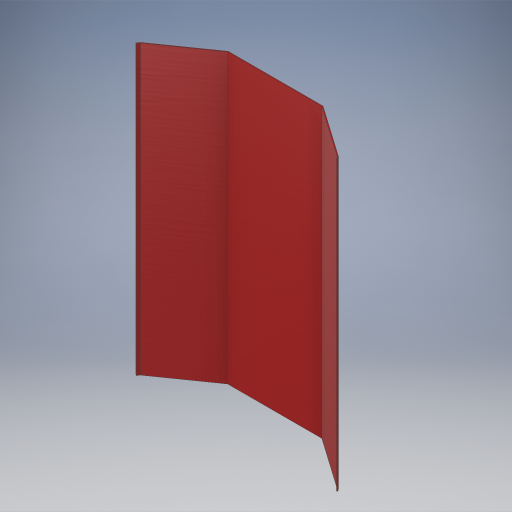
# Autodesk Inventor part: Gummi Matte
Saved by Autodesk Inventor 2023.2 (Build 272271000, 271)
## iProperties
Created: 2023-02-05
Part Number: Gummi Matte
Material: Gummi
Document SubType Name: Modeling
Designer: Raoul Messerli
Density: 0.93 g/cm^3
Appearance: Gummi - Schwarz
Author: Raoul Messerli
Autodesk Inventor part; units mm, degrees
ref_plane "YZ Plane" through (0, 0, 0) normal (1, 0, 0) x (0, 1, 0)
ref_plane "XZ Plane" through (0, 0, 0) normal (0, 1, 0) x (-1, 0, 0)
ref_plane "XY Plane" through (0, 0, 0) normal (0, 0, 1) x (1, 0, 0)
sketch "Skizze1" plane through (0, 0, 0) normal (0, 0, 1) x (1, 0, 0)
  line L0 (0, 0) -> (148.3505, 0)
  line L1 (0, 0) -> (-148.3505, 0)
  line L2 (-148.3505, 0) -> (-310.097, -113.2561)
  line L3 (148.3505, 0) -> (310.097, -113.2561)
  line L4 (310.097, -113.2561) -> (315.8328, -121.4476)
  line L5 (-310.097, -113.2561) -> (-315.8328, -121.4476)
  line L6 (-313.3753, -123.1684) -> (-307.9429, -115.4102)
  line L7 (-307.9429, -115.4102) -> (-147.4046, -3)
  line L8 (-147.4046, -3) -> (0, -3)
  line L9 (0, -3) -> (147.4046, -3)
  line L10 (147.4046, -3) -> (307.9429, -115.4102)
  line L11 (307.9429, -115.4102) -> (313.3753, -123.1684)
  line L12 (-315.8328, -121.4476) -> (-313.3753, -123.1684)
  line L13 (315.8328, -121.4476) -> (313.3753, -123.1684)
  dimension "d0" = 145
  dimension "d1" = 160
  dimension "d2" = 145
  dimension "d3" = 160
  dimension "d4" = 197.456
  dimension "d5" = 296.701
  dimension "d6" = 10
  dimension "d7" = 3
  constraints: 28 end point, 3 equal length, 2 horizontal, 5 other
  measures "d0" angle of L1 L2
  measures "d1" angle of L2 L5
  measures "d2" angle of L3 L0
  measures "d3" angle of L4 L3
  measures "d4" distance of L1.end L2.end
  measures "d5" distance of L0.end L1.end
  measures "d6" distance of L2.end L5.end
  measures "d7" distance between parallel lines of L5 L6
extrude "Extrusion1" add sketch "Skizze1" along normal blind 900
